mount_farm (Autodesk Fusion 360 design; units mm, degrees)
Autodesk Fusion 360 part; units mm, degrees
sketch "Sketch1" plane through (0, 0, 0) normal (0, 0, 1) x (1, 0, 0)
  line L0 (0, 0) -> (20, 0)
  line L1 (20, 0) -> (20, 20)
  line L2 (20, 20) -> (0, 20)
  line L3 (0, 20) -> (0, 0)
  dimension "d1" = 20
  dimension "d2" = 20
  constraint horizontal L0
  constraint vertical L1
  constraint horizontal L2
  constraint vertical L3
  constraint coincident L0.start L3.end
  measures "d1" distance of L0.start L0.end
  measures "d2" distance of L0.start L2.end
extrude "Extrude1" add sketch "Sketch1" along normal blind 3
sketch "Sketch2" plane through (0, 0, 3) normal (0, 0, 1) x (-1, 0, 0)
  line L0 (0, -20) -> (0, 0)
  line L1 (0, 0) -> (-20, 0)
  line L2 (-20, 0) -> (-20, -20)
  line L3 (-20, -20) -> (0, -20)
  line L4 (0, 0) -> (-20, 0)
  line L5 (-20, 0) -> (-20, -3)
  line L6 (-20, -3) -> (0, -3)
  line L7 (0, -3) -> (0, 0)
  dimension "d5" = 20
  dimension "d6" = 3
  constraint horizontal L4
  constraint vertical L5
  constraint horizontal L6
  constraint vertical L7
  constraint coincident L0.end L1.start
  measures "d5" distance of L0.end L1.end
  measures "d6" distance of L0.end L6.end
extrude "Extrude2" add sketch "Sketch2" along normal blind 17 contours L0 L1 L2 L4 L5 L6 L7
sketch "Sketch3" plane through (0, 0, 3) normal (0, 0, 1) x (-1, 0, 0)
  line L0 (0, -3) -> (-20, -3)
  line L1 (-20, -3) -> (-20, -20)
  line L2 (-20, -20) -> (0, -20)
  line L3 (0, -20) -> (0, -3)
  line L4 (-10, -20) -> (-10, -3) construction
  point P0 (-10, -11.5)
  constraint midpoint L2 L4.start
  constraint midpoint L0 L4.end
  constraint midpoint L4 P0
hole "Hole1" at (10, 11.5, 3) direction (0, 0, -1) diameter 3.4 depth 10 tip angle 180 countersink diameter 6.3 countersink angle 90
fillet "Fillet1" radius 4 1 edges at (10, 3, 3)
